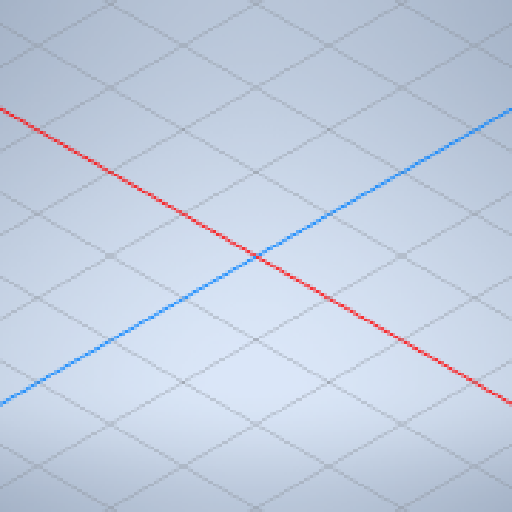
# Autodesk Inventor part: 电气支架_2
Saved by Autodesk Inventor 2025.1 (Build 291241000, 241)
## iProperties
Created: 2025-09-04
Part Number: 电气支架_2
Material: 常规
Document SubType Name: Modeling
Designer: Piw
Density: 1 g/cm^3
Appearance: 默认
Author: Piw
Autodesk Inventor part; units mm, degrees
ref_plane "YZ Plane" through (0, 0, 0) normal (1, 0, 0) x (0, 1, 0)
ref_plane "XZ Plane" through (0, 0, 0) normal (0, 1, 0) x (-1, 0, 0)
ref_plane "XY Plane" through (0, 0, 0) normal (0, 0, 1) x (1, 0, 0)
ref_plane "工作平面1" through (19.3371, -7.6679, 114.989) normal (-1, 0, 0) x (0, -1, 0)
sketch "草图1" plane through (19.3371, -7.6679, 114.989) normal (-1, 0, 0) x (0, -1, 0)
  circle A0 centre (20, 75) radius 2.1
  circle A1 centre (20, 90) radius 2.1
  circle A2 centre (20, 60) radius 2.1
  circle A3 centre (8, 60) radius 2.1
  circle A4 centre (8, 90) radius 2.1
  line L0 (0, 0) -> (0, 214)
  circle A5 centre (12.0096, 5) radius 2.1
  circle A6 centre (25, 12.5) radius 2.1
  circle A7 centre (37.9904, 5) radius 2.1
  circle A8 centre (20, 75) radius 2.1
  circle A9 centre (20, 90) radius 2.1
  circle A10 centre (20, 60) radius 2.1
  circle A11 centre (8, 90) radius 2.1
  circle A12 centre (8, 60) radius 2.1
  circle A13 centre (15.7729, 200.5) radius 2.1
  circle A14 centre (28.7632, 208) radius 2.1
  circle A15 centre (28.7632, 178) radius 2.1
  circle A16 centre (15.7729, 185.5) radius 2.1
  circle A17 centre (41.7536, 200.5) radius 2.1
  circle A18 centre (41.7536, 185.5) radius 2.1
  circle A19 centre (28.7632, 193) radius 7.5
  arc A20 (48.2862, 199.5655) -> (25.6285, 214) centre (25.6285, 189) ccw
  line L1 (25.6285, 214) -> (0, 214)
  line L2 (0, 0) -> (0, 214)
  line L3 (0, 0) -> (64, 0)
  line L4 (64, 0) -> (64, 23)
  line L5 (66.8284, 25) -> (64, 23)
  line L6 (66.8284, 25) -> (70, 25)
  line L7 (70, 25) -> (70, 147.4576)
  arc A21 (70, 147.4576) -> (67.6577, 158.0231) centre (45, 147.4576) ccw
  line L8 (67.6577, 158.0231) -> (48.2862, 199.5655)
  circle A22 centre (64.4234, 100.25) radius 2.1
  circle A23 centre (37.5766, 49.75) radius 2.1
  circle A24 centre (64.4234, 65.25) radius 2.1
  circle A25 centre (37.5766, 100.25) radius 2.1
  circle A26 centre (64.4234, 84.75) radius 2.1
  circle A27 centre (51, 42) radius 2.1
  circle A28 centre (64.4234, 49.75) radius 2.1
  circle A29 centre (51, 108) radius 2.1
  circle A30 centre (33.7425, 67) radius 3.25
  circle A31 centre (59, 75) radius 3.25
  circle A32 centre (33.7425, 83) radius 3.25
  circle A33 centre (50, 75) radius 3.25
  circle A34 centre (41, 75) radius 3.25
  line L9 (0, 47.65) -> (28, 47.65)
  line L10 (28, 47.65) -> (28, 102.35)
  line L11 (28, 102.35) -> (0, 102.35)
  line L12 (0, 102.35) -> (0, 47.65)
  point P0 (-7.6679, -114.989)
  point P1 (0, 102.35)
  point P2 (0, 47.65)
extrude "拉伸1" add sketch "草图1" along normal blind 7 contours L0 L11 L10 L9
sketch "草图2" plane through (19.3371, -35.6679, 217.339) normal (0, 0, 1) x (1, 0, 0)
  line L0 (-6, -42) -> (-116, -42) projected
  line L1 (-6, -42) -> (-43, -42)
  line L2 (-43, -42) -> (-43, -14)
  line L3 (-43, -14) -> (-6, -14)
  line L4 (-6, -14) -> (-6, -42)
  line L5 (-48, -3.4068) -> (-48, -11.4068) projected
  line L6 (-47, -3.4068) -> (-47, 27) projected
  line L7 (0, 0) -> (-7, 0) projected
  line L8 (-7, 0) -> (-47, -3.4068)
  line L9 (-47, -3.4068) -> (-47, -42)
  line L10 (0, 0) -> (0, -3)
  line L11 (0, -3) -> (-44, -6.7475)
  line L12 (-44, -6.7475) -> (-44, -42)
  point P0 (-19.3371, 35.6679)
  dimension "d3" = 37
  dimension "d4" = 28
  dimension "d5" = 3
  dimension "d6" = 3
  constraints: 18 end point, 3 parallel, 3 perpendicular, 2 point on line, 1 horizontal, 1 vertical
  measures "d3" distance of L2.end L3.end
  measures "d4" distance of L1.end L2.end
  measures "d5" distance of L7.start L10.end
  measures "d6" distance between parallel lines of L9 L12
extrude "拉伸2" add sketch "草图2" against normal up to surface (54.7 mm away) contours L0 L9 L8 L7 L10 L11 L12
chamfer "倒角1" distance 2 angle 45 1 edges at (-24.6629, -42.4154, 189.989)
sketch "草图3" plane through (-24.6629, -77.6679, 217.339) normal (1, 0, 0) x (0, 0, -1)
  line L0 (0, 0) -> (0, 33.2525) projected
  line L1 (0, 0) -> (80, 0)
  line L2 (80, 0) -> (80, 4)
  line L3 (80, 4) -> (0, 4)
  line L4 (0, 4) -> (0, 0)
  point P0 (217.339, 77.6679)
  point P1 (0, 4)
  dimension "d12" = 80
  dimension "d13" = 4
  constraints: 8 end point, 2 parallel, 1 horizontal, 1 perpendicular
  measures "d12" distance of L3.end L2.end
  measures "d13" distance between parallel lines of L1 L3
extrude "拉伸3" add sketch "草图3" along normal blind 35
chamfer "倒角2" distance 2 angle 45 8 edges at (10.3371, -75.6679, 217.339) (10.3371, -75.6679, 137.339) (-27.6629, -39.0748, 189.989) (-24.6629, -75.6679, 137.339) (-24.6629, -75.6679, 162.639) (12.3371, -35.6679, 189.989) (19.3371, -38.6679, 189.989) (-27.6629, -77.6679, 189.989)
sketch "草图4" plane through (-24.6629, -73.6679, 217.339) normal (0, 1, 0) x (1, 0, 0)
  line L0 (2, 80) -> (33, 80) projected
  line L1 (19, 80) -> (19, -0.4467) construction
  line L2 (0, 78) -> (0, 56.7) projected
  line L3 (44, -44.0038) -> (44, 260.8962) projected
  circle A0 centre (19, 69) radius 1.9
  circle A1 centre (19, 7) radius 1.9
  point P0 (24.6629, 217.339)
  dimension "d19" = 19
  dimension "d20" = 25
  dimension "d21" = 3.8
  dimension "d22" = 3.8
  dimension "d23" = 62
  dimension "d24" = 11
  constraints: 3 point on line, 2 centre point, 2 end point, 1 vertical
  measures "d19" distance between parallel lines of L2 L1
  measures "d20" distance between parallel lines of L3 L1
  measures "d21" diameter of A0
  measures "d22" diameter of A1
  measures "d23" distance of A0.centre A1.centre
  measures "d24" distance from line of L0 A0.centre
extrude "拉伸4" cut sketch "草图4" against normal blind 35
